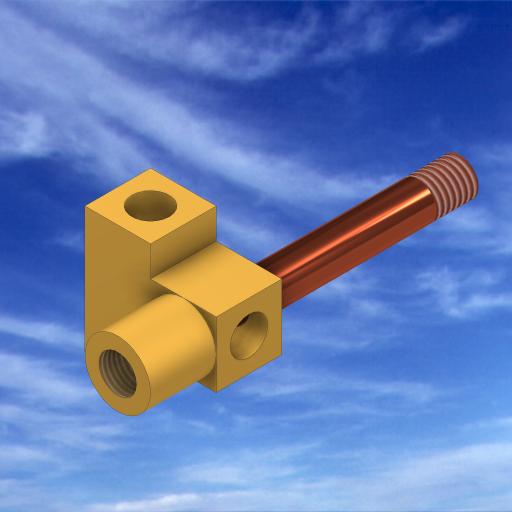
# Autodesk Inventor part: HUDSON-1-45
Saved by Autodesk Inventor 2024.2 (Build 282272000, 272)
## iProperties
Created: 2024-10-10
Part Number: HUDSON-1-45
Material: Generic
Document SubType Name: Modeling
Designer: Precisión-05
Density: 1 g/cm^3
Appearance: Default
Author: Precisión-05
Autodesk Inventor part; units mm, degrees
ref_plane "YZ Plane" through (0, 0, 0) normal (1, 0, 0) x (0, 1, 0)
ref_plane "XZ Plane" through (0, 0, 0) normal (0, 1, 0) x (-1, 0, 0)
ref_plane "XY Plane" through (0, 0, 0) normal (0, 0, 1) x (1, 0, 0)
sketch "Sketch1" plane through (0, 0, 0) normal (0, 0, 1) x (1, 0, 0)
  line L0 (-7, 7) -> (7, 7)
  line L1 (7, 7) -> (7, -7)
  line L2 (7, -7) -> (-7, -7)
  line L3 (-7, -7) -> (-7, 7)
  line L4 (-7, 7) -> (7, -7) construction
  line L5 (7, 7) -> (-7, -7) construction
  point P0 (0, 0)
  dimension "d0" = 14
  dimension "d1" = 14
  constraints: 12 end point, 2 midpoint, 2 parallel, 1 horizontal, 1 perpendicular
  measures "d0" distance of L1.end L2.end
  measures "d1" distance of L0.end L1.end
extrude "Extrusion1" add sketch "Sketch1" along normal blind 28
sketch "Sketch2" plane through (7, -7, 0) normal (1, 0, 0) x (0, 0, -1)
  line L0 (-28, 0) -> (-28, 14) projected
  line L1 (-28, 14) -> (-14, 14)
  line L2 (-14, 14) -> (-14, 0)
  line L3 (-14, 0) -> (-28, 0)
  line L4 (-28, 0) -> (-28, 14)
  point P0 (0, 7)
  dimension "d4" = 14
  dimension "d5" = 14
  constraints: 8 end point, 2 parallel, 1 horizontal, 1 perpendicular
  measures "d4" distance of L2.end L3.end
  measures "d5" distance of L1.end L2.end
extrude "Extrusion2" add sketch "Sketch2" along normal blind 14
sketch "Sketch3" plane through (21, -7, 0) normal (1, 0, 0) x (0, 0, -1)
  line L0 (-14, 0) -> (-14, 14) projected
  line L1 (-14, 14) -> (-28, 14) projected
  line L2 (-28, 14) -> (-28, 0) projected
  line L3 (-28, 0) -> (-14, 0) projected
  line L4 (-28, 14) -> (-14, 14)
  line L5 (-14, 14) -> (-14, 0)
  line L6 (-14, 0) -> (-28, 0)
  line L7 (-28, 0) -> (-28, 14)
  point P0 (0, 7)
  point P1 (-21, 7)
  constraints: 8 end point, 2 parallel, 1 horizontal, 1 perpendicular
hole "Hole1" at (21, 0, 21) direction (-1, 0, 0) diameter 8 depth 25
sketch "Sketch4" plane through (0, 0, 0) normal (0, 0, -1) x (-1, 0, 0)
  line L0 (7, -7) -> (-7, -7) projected
  line L1 (7, 7) -> (7, -7) projected
  line L2 (-7, 7) -> (7, 7) projected
  line L3 (-7, -7) -> (-7, 7) projected
  point P0 (0, 0)
  point P1 (0, 0)
  constraints: 1 coincident
sketch "Sketch5" plane through (-7, 7, 0) normal (0, 1, 0) x (1, 0, 0)
  line L0 (14, 0) -> (0, 0) projected
  line L1 (0, 0) -> (0, -28) projected
  line L2 (0, -28) -> (28, -28) projected
  line L3 (28, -14) -> (28, -28) projected
  line L4 (14, -14) -> (28, -14) projected
  line L5 (14, 0) -> (14, -14) projected
  line L6 (14, -14) -> (28, -14)
  line L7 (28, -14) -> (28, -28)
  line L8 (28, -28) -> (14, -28)
  line L9 (14, -28) -> (14, -14)
  circle A0 centre (21, -21) radius 4
  point P0 (7, 0)
  dimension "d23" = 8
  constraints: 8 end point, 2 parallel, 1 centre point, 1 coincident, 1 horizontal, 1 perpendicular
  measures "d23" diameter of A0
extrude "Extrusion3" add sketch "Sketch5" along normal blind 45 contours A0
thread "Thread1" size "M8x1.25" class "6g" standard "ANSI Metric M Profile" length 45 offset 36
sketch "Sketch6" plane through (14, 52, 21) normal (0, 1, 0) x (1, 0, 0)
  circle A0 centre (0, 0) radius 4 projected
  point P0 (-14, 21)
  constraints: 1 coincident
hole "Hole3" at (14, 52, 21) direction (0, -1, 0) diameter 6 depth 50 tip angle 118
sketch "Sketch7" plane through (-7, -7, 0) normal (0, -1, 0) x (1, 0, 0)
  line L0 (28, 28) -> (28, 14) projected
  line L1 (14, 14) -> (28, 14) projected
  line L2 (28, 28) -> (14, 28)
  line L3 (14, 28) -> (14, 14)
  line L4 (14, 14) -> (28, 14)
  line L5 (28, 14) -> (28, 28)
  circle A0 centre (21, 21) radius 3 projected
  circle A1 centre (21, 21) radius 7
  circle A2 centre (21, 21) radius 4 projected
  circle A3 centre (21, 21) radius 4
  line L6 (21, 21) -> (0, 21)
  line L7 (0, 0) -> (0, 28) projected
  line L8 (0, 21) -> (0, 34.5)
  line L9 (0, 34.5) -> (0, 21)
  line L10 (0, 21) -> (0, 7.5)
  point P0 (7, 0)
  dimension "d35" = 14
  dimension "d36" = 8
  dimension "d37" = 13.5
  dimension "d38" = 13.5
  constraints: 16 end point, 3 equal length, 2 centre point, 2 coincident, 2 horizontal, 2 perpendicular, 2 point on line
  measures "d35" diameter of A1
  measures "d36" diameter of A3
  measures "d37" distance of L6.end L8.end
  measures "d38" distance of L6.end L10.end
sketch "Sketch8" plane through (0, 0, 0) normal (0, 0, -1) x (-1, 0, 0)
  line L0 (7, -7) -> (-7, -7) projected
  line L1 (7, 7) -> (7, -7) projected
  line L2 (-7, -7) -> (7, -7)
  line L3 (7, -7) -> (7, 7)
  line L4 (7, 7) -> (-7, 7)
  line L5 (-7, 7) -> (-7, -7)
  point P0 (0, 0)
  constraints: 8 end point, 2 parallel, 1 horizontal, 1 perpendicular
extrude "Extrusion4" cut sketch "Sketch8" against normal blind 7.5
sketch "Sketch9" plane through (0, 0, 28) normal (0, 0, 1) x (1, 0, 0)
  line L0 (-7, 7) -> (21, 7) projected
  line L1 (-7, 7) -> (7, 7)
  line L2 (7, 7) -> (7, -7)
  line L3 (7, -7) -> (-7, -7)
  line L4 (-7, -7) -> (-7, 7)
  point P0 (0, 0)
  dimension "d41" = 14
  dimension "d42" = 14
  constraints: 8 end point, 2 parallel, 1 horizontal, 1 perpendicular
  measures "d41" distance of L2.end L3.end
  measures "d42" distance of L1.end L2.end
extrude "Extrusion5" add sketch "Sketch9" along normal blind 6.5
hole "Hole4" at (0, 0, 0) direction (0, 0, 1) diameter 8 end through all
extrude "Extrusion6" add sketch "Sketch7" along normal blind 14 contours A1
thread "Thread2" size "M8x1" class "6H" standard "ANSI Metric M Profile" length 45
sketch "Sketch10" plane through (14, -7, 21) normal (0, -1, 0) x (1, 0, 0)
  circle A0 centre (0, 0) radius 4 projected
  point P0 (-14, -21)
  constraints: 1 coincident
hole "Hole5" at (14, -7, 21) direction (0, 1, 0) diameter 5 depth 8
body "Solid1"
